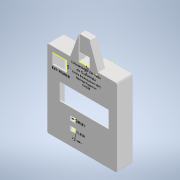
# Autodesk Inventor part: Cubierta SUperior
Saved by Autodesk Inventor 2021 (Build 250183000, 183)
## iProperties
Created: 2021-08-03
Part Number: Cubierta SUperior
Material: Generic
Document SubType Name: Modeling
Designer: Admin
Density: 1 g/cm^3
Appearance: Default
Author: Admin
Autodesk Inventor part; units mm, degrees
(part 1 of 3)
ref_plane "YZ Plane" through (0, 0, 0) normal (1, 0, 0) x (0, 1, 0)
ref_plane "XZ Plane" through (0, 0, 0) normal (0, 1, 0) x (-1, 0, 0)
ref_plane "XY Plane" through (0, 0, 0) normal (0, 0, 1) x (1, 0, 0)
sketch "Sketch1" plane through (0, 0, 0) normal (0, 0, 1) x (1, 0, 0)
  line L0 (-67.4504, -0.753) -> (-67.4504, -101.753) construction
  line L1 (24.2036, -1.253) -> (24.2036, -101.253) construction
  line L2 (24.2036, -101.253) -> (-64.9504, -101.253) construction
  line L3 (-64.9504, -101.253) -> (-64.9504, -1.253) construction
  line L4 (-64.9504, -1.253) -> (24.2036, -1.253) construction
  arc A0 (-65.4504, 1.247) -> (-67.4504, -0.753) centre (-65.4504, -0.753) ccw projected
  line L5 (-67.4504, -0.753) -> (-67.4504, -101.753) projected
  arc A1 (-67.4504, -101.753) -> (-65.4504, -103.753) centre (-65.4504, -101.753) ccw projected
  line L6 (-65.4504, -103.753) -> (26.7036, -103.753) projected
  line L7 (26.7036, -103.753) -> (26.7036, -0.753) projected
  arc A2 (26.7036, -0.753) -> (24.7036, 1.247) centre (24.7036, -0.753) ccw projected
  line L8 (24.7036, 1.247) -> (-65.4504, 1.247) projected
  line L9 (-52.1604, -58.503) -> (17.2396, -58.503) projected
  line L10 (17.2396, -58.503) -> (17.2396, -34.603) projected
  line L11 (17.2396, -34.603) -> (-52.1604, -34.603) projected
  line L12 (-52.1604, -34.603) -> (-52.1604, -58.503) projected
  line L13 (13.9003, -56.603) -> (-48.821, -56.603) projected
  arc A3 (14.3003, -57.003) -> (13.9003, -56.603) centre (13.9003, -57.003) ccw projected
  line L14 (14.3003, -57.203) -> (14.3003, -57.003) projected
  arc A4 (13.9003, -57.603) -> (14.3003, -57.203) centre (13.9003, -57.203) ccw projected
  line L15 (-48.821, -57.603) -> (13.9003, -57.603) projected
  arc A5 (-49.221, -57.203) -> (-48.821, -57.603) centre (-48.821, -57.203) ccw projected
  line L16 (-49.221, -57.003) -> (-49.221, -57.203) projected
  arc A6 (-48.821, -56.603) -> (-49.221, -57.003) centre (-48.821, -57.003) ccw projected
  line L17 (-49.221, -35.903) -> (-49.221, -36.103) projected
  arc A7 (-48.821, -35.503) -> (-49.221, -35.903) centre (-48.821, -35.903) ccw projected
  line L18 (13.9003, -35.503) -> (-48.821, -35.503) projected
  arc A8 (14.3003, -35.903) -> (13.9003, -35.503) centre (13.9003, -35.903) ccw projected
  line L19 (14.3003, -36.103) -> (14.3003, -35.903) projected
  arc A9 (13.9003, -36.503) -> (14.3003, -36.103) centre (13.9003, -36.103) ccw projected
  line L20 (-48.821, -36.503) -> (13.9003, -36.503) projected
  arc A10 (-49.221, -36.103) -> (-48.821, -36.503) centre (-48.821, -36.103) ccw projected
  line L21 (13.2396, -39.653) -> (-48.1604, -39.653) projected
  arc A11 (14.7396, -41.153) -> (13.2396, -39.653) centre (13.2396, -41.153) ccw projected
  line L22 (14.7396, -51.953) -> (14.7396, -41.153) projected
  arc A12 (13.2396, -53.453) -> (14.7396, -51.953) centre (13.2396, -51.953) ccw projected
  line L23 (-48.1604, -53.453) -> (13.2396, -53.453) projected
  arc A13 (-49.6604, -51.953) -> (-48.1604, -53.453) centre (-48.1604, -51.953) ccw projected
  line L24 (-49.6604, -41.153) -> (-49.6604, -51.953) projected
  arc A14 (-48.1604, -39.653) -> (-49.6604, -41.153) centre (-48.1604, -41.153) ccw projected
  arc A15 (-67.9504, 3.747) -> (-69.9504, 1.747) centre (-67.9504, 1.747) ccw projected
  line L25 (-67.9504, 3.747) -> (27.2036, 3.747) projected
  arc A16 (29.2036, 1.747) -> (27.2036, 3.747) centre (27.2036, 1.747) ccw projected
  line L26 (29.2036, 1.747) -> (29.2036, -104.253) projected
  arc A17 (27.2036, -106.253) -> (29.2036, -104.253) centre (27.2036, -104.253) ccw projected
  line L27 (27.2036, -106.253) -> (-67.9504, -106.253) projected
  arc A18 (-69.9504, -104.253) -> (-67.9504, -106.253) centre (-67.9504, -104.253) ccw projected
  line L28 (-69.9504, -104.253) -> (-69.9504, 1.747) projected
  circle A19 centre (-54.7104, -61.153) radius 1.7 construction
  circle A20 centre (-54.7104, -30.653) radius 1.7 construction
  circle A21 centre (19.7896, -61.153) radius 1.7 construction
  circle A22 centre (19.7896, -30.653) radius 1.7 construction
  line L29 (-64.9504, -101.253) -> (-64.9504, -1.253) projected
  line L30 (-64.9504, -1.253) -> (24.2036, -1.253) projected
  line L31 (24.2036, -1.253) -> (24.2036, -101.253) projected
  line L32 (24.2036, -101.253) -> (-64.9504, -101.253) projected
  line L33 (-74.9504, -109.253) -> (-74.9504, 6.747)
  arc A23 (-74.9504, -109.253) -> (-72.9504, -111.253) centre (-72.9504, -109.253) ccw
  line L34 (32.2036, -111.253) -> (-72.9504, -111.253)
  arc A24 (32.2036, -111.253) -> (34.2036, -109.253) centre (32.2036, -109.253) ccw
  line L35 (34.2036, 6.747) -> (34.2036, -109.253)
  arc A25 (34.2036, 6.747) -> (32.2036, 8.747) centre (32.2036, 6.747) ccw
  line L36 (-72.9504, 8.747) -> (32.2036, 8.747)
  arc A26 (-72.9504, 8.747) -> (-74.9504, 6.747) centre (-72.9504, 6.747) ccw
  point P0 (0, 0)
  constraints: 8 end point, 8 point on circle, 4 centre point, 2 horizontal, 2 vertical, 16 other
extrude "Extrusion1" add sketch "Sketch1" along normal blind 22.5 contours L25 A16 L26 A17 L27 A18 L28 A15
sketch "Sketch2" plane through (0, 0, 22.5) normal (0, 0, 1) x (1, 0, 0)
  line L0 (-52.1604, -58.503) -> (17.2396, -58.503) projected
  line L1 (17.2396, -58.503) -> (17.2396, -34.603) projected
  line L2 (17.2396, -34.603) -> (-52.1604, -34.603) projected
  line L3 (-52.1604, -34.603) -> (-52.1604, -58.503) projected
  line L4 (13.9003, -56.603) -> (-48.821, -56.603) projected
  arc A0 (14.3003, -57.003) -> (13.9003, -56.603) centre (13.9003, -57.003) ccw projected
  line L5 (14.3003, -57.203) -> (14.3003, -57.003) projected
  arc A1 (13.9003, -57.603) -> (14.3003, -57.203) centre (13.9003, -57.203) ccw projected
  line L6 (-48.821, -57.603) -> (13.9003, -57.603) projected
  arc A2 (-49.221, -57.203) -> (-48.821, -57.603) centre (-48.821, -57.203) ccw projected
  line L7 (-49.221, -57.003) -> (-49.221, -57.203) projected
  arc A3 (-48.821, -56.603) -> (-49.221, -57.003) centre (-48.821, -57.003) ccw projected
  line L8 (-49.221, -35.903) -> (-49.221, -36.103) projected
  arc A4 (-48.821, -35.503) -> (-49.221, -35.903) centre (-48.821, -35.903) ccw projected
  line L9 (13.9003, -35.503) -> (-48.821, -35.503) projected
  arc A5 (14.3003, -35.903) -> (13.9003, -35.503) centre (13.9003, -35.903) ccw projected
  line L10 (14.3003, -36.103) -> (14.3003, -35.903) projected
  arc A6 (13.9003, -36.503) -> (14.3003, -36.103) centre (13.9003, -36.103) ccw projected
  line L11 (-48.821, -36.503) -> (13.9003, -36.503) projected
  arc A7 (-49.221, -36.103) -> (-48.821, -36.503) centre (-48.821, -36.103) ccw projected
  line L12 (13.2396, -39.653) -> (-48.1604, -39.653) projected
  arc A8 (14.7396, -41.153) -> (13.2396, -39.653) centre (13.2396, -41.153) ccw projected
  line L13 (14.7396, -51.953) -> (14.7396, -41.153) projected
  arc A9 (13.2396, -53.453) -> (14.7396, -51.953) centre (13.2396, -51.953) ccw projected
  line L14 (-48.1604, -53.453) -> (13.2396, -53.453) projected
  arc A10 (-49.6604, -51.953) -> (-48.1604, -53.453) centre (-48.1604, -51.953) ccw projected
  line L15 (-49.6604, -41.153) -> (-49.6604, -51.953) projected
  arc A11 (-48.1604, -39.653) -> (-49.6604, -41.153) centre (-48.1604, -41.153) ccw projected
  line L16 (27.2036, 3.747) -> (-67.9504, 3.747) projected
  arc A12 (-67.9504, 3.747) -> (-69.9504, 1.747) centre (-67.9504, 1.747) ccw projected
  line L17 (-69.9504, 1.747) -> (-69.9504, -104.253) projected
  arc A13 (-69.9504, -104.253) -> (-67.9504, -106.253) centre (-67.9504, -104.253) ccw projected
  line L18 (-67.9504, -106.253) -> (27.2036, -106.253) projected
  arc A14 (27.2036, -106.253) -> (29.2036, -104.253) centre (27.2036, -104.253) ccw projected
  line L19 (29.2036, -104.253) -> (29.2036, 1.747) projected
  arc A15 (29.2036, 1.747) -> (27.2036, 3.747) centre (27.2036, 1.747) ccw projected
  line L20 (-35.8504, -70.273) -> (-35.8504, -73.173) construction
  line L21 (-35.8504, -73.173) -> (-31.8504, -73.173) construction
  line L22 (-31.8504, -73.173) -> (-31.8504, -70.273) construction
  line L23 (-31.8504, -70.273) -> (-35.8504, -70.273) construction
  circle A16 centre (-33.8504, -71.723) radius 0.875 construction
  line L24 (-31.8504, -85.773) -> (-31.8504, -82.873) construction
  line L25 (-31.8504, -82.873) -> (-35.8504, -82.873) construction
  line L26 (-35.8504, -82.873) -> (-35.8504, -85.773) construction
  line L27 (-35.8504, -85.773) -> (-31.8504, -85.773) construction
  circle A17 centre (-33.8504, -84.323) radius 0.875 construction
  line L28 (-37.3504, -68.773) -> (-37.3504, -74.673)
  line L29 (-37.3504, -74.673) -> (-30.3504, -74.673)
  line L30 (-30.3504, -74.673) -> (-30.3504, -68.773)
  line L31 (-30.3504, -68.773) -> (-37.3504, -68.773)
  line L32 (-37.3504, -81.373) -> (-30.3504, -81.373)
  line L33 (-30.3504, -81.373) -> (-30.3504, -87.273)
  line L34 (-30.3504, -87.273) -> (-37.3504, -87.273)
  line L35 (-37.3504, -87.273) -> (-37.3504, -81.373)
  point P0 (0, 0)
  dimension "d4" = 1.5
  dimension "d5" = 1.5
  constraints: 16 end point, 6 other
  measures "d4" distance between parallel lines of L31 L23
  measures "d5" distance between parallel lines of L32 L25
sketch "Sketch3" plane through (-67.9504, -106.253, 0) normal (0, -1, 0) x (1, 0, 0)
  line L0 (0, 0) -> (95.154, 0) construction
  line L1 (1.5, 20) -> (95.654, 20) construction
  line L2 (0, 22.5) -> (95.154, 22.5) construction
  line L3 (47.577, 22.5) -> (47.577, 0) construction
  line L4 (39.5436, 0) -> (55.4643, 0)
  line L5 (55.4643, 0) -> (55.4643, 6.6011)
  line L6 (55.4643, 6.6011) -> (39.5436, 6.6011)
  line L7 (39.5436, 6.6011) -> (39.5436, 0)
  line L8 (0, 0) -> (0, 22.5) projected
  point P0 (67.9504, 0)
  dimension "d6" = 39.5436
  dimension "d7" = 15.9207
  dimension "d8" = 13.3989
  constraints: 10 end point, 2 midpoint, 2 parallel, 1 horizontal, 1 perpendicular, 1 point on line
  measures "d6" distance between parallel lines of L8 L7
  measures "d7" distance of L5.end L6.end
  measures "d8" distance between parallel lines of L1 L6
extrude "Extrusion3" cut sketch "Sketch3" against normal blind 3
sketch "Sketch4" plane through (0, 0, 22.5) normal (0, 0, 1) x (1, 0, 0)
  line L0 (27.2036, 3.747) -> (-67.9504, 3.747) projected
  arc A0 (-67.9504, 3.747) -> (-69.9504, 1.747) centre (-67.9504, 1.747) ccw projected
  line L1 (-69.9504, 1.747) -> (-69.9504, -104.253) projected
  arc A1 (-69.9504, -104.253) -> (-67.9504, -106.253) centre (-67.9504, -104.253) ccw projected
  line L2 (-67.9504, -106.253) -> (27.2036, -106.253) projected
  arc A2 (27.2036, -106.253) -> (29.2036, -104.253) centre (27.2036, -104.253) ccw projected
  line L3 (29.2036, -104.253) -> (29.2036, 1.747) projected
  arc A3 (29.2036, 1.747) -> (27.2036, 3.747) centre (27.2036, 1.747) ccw projected
  line L4 (-65.4504, 1.247) -> (24.7036, 1.247) projected
  arc A4 (26.7036, -0.753) -> (24.7036, 1.247) centre (24.7036, -0.753) ccw projected
  line L5 (26.7036, -0.753) -> (26.7036, -103.753) projected
  line L6 (26.7036, -103.753) -> (-65.4504, -103.753) projected
  arc A5 (-67.4504, -101.753) -> (-65.4504, -103.753) centre (-65.4504, -101.753) ccw projected
  line L7 (-67.4504, -101.753) -> (-67.4504, -0.753) projected
  arc A6 (-65.4504, 1.247) -> (-67.4504, -0.753) centre (-65.4504, -0.753) ccw projected
  point P0 (0, 0)
extrude "Extrusion5" add sketch "Sketch4" against normal blind 2 contours L4 A4 L5 L6 A5 L7 A6
extrude "Extrusion4" cut sketch "Sketch2" against normal blind 12.25 contours L3 L2 L1 L0 | A0 L5 A1 L6 A2 L7 A3 L4 | A4 L9 A5 L10 A6 L11 A7 L8 | A8 L13 A9 L14 A10 L15 A11 L12 | L31 L30 L29 L28 | L32 L33 L34 L35
sketch "Sketch5" plane through (-67.9504, 3.747, 0) normal (0, 1, 0) x (1, 0, 0)
  point P0 (67.9504, 0)
sketch "Sketch6" plane through (-67.9504, 3.747, 0) normal (0, 1, 0) x (1, 0, 0)
  line L0 (58.24, -22.5) -> (42.74, -22.5)
  line L1 (42.74, -22.5) -> (42.74, -12.5)
  line L2 (42.74, -12.5) -> (58.24, -12.5)
  line L3 (58.24, -12.5) -> (58.24, -22.5)
  line L4 (15.79, -22.5) -> (85.19, -22.5) projected
  point P0 (67.9504, 0)
  point P1 (50.49, -22.5)
  point P2 (50.49, -22.5)
  dimension "d15" = 15.5
  dimension "d16" = 10
  constraints: 8 end point, 3 midpoint, 2 parallel, 1 coincident, 1 horizontal, 1 perpendicular
  measures "d15" distance of L1.end L2.end
  measures "d16" distance of L0.end L1.end
extrude "Extrusion6" add sketch "Sketch6" along normal blind 33
sketch "Sketch7" plane through (0, 0, 22.5) normal (0, 0, 1) x (1, 0, 0)
  line L0 (-25.2104, 36.747) -> (-9.7104, 36.747) projected
  line L1 (-9.7104, 36.747) -> (2.3007, 3.747)
  line L2 (27.2036, 3.747) -> (-67.9504, 3.747) projected
  line L3 (-25.2104, 3.747) -> (-25.2104, 36.747) projected
  line L4 (-25.2104, 36.747) -> (-37.2214, 3.747)
  line L5 (-25.2104, 3.747) -> (-67.9504, 3.747) projected
  line L6 (2.3007, 3.747) -> (-37.2214, 3.747)
  line L7 (-9.7104, 3.747) -> (-9.7104, 36.747) projected
  point P0 (0, 0)
  point P1 (-37.2214, 3.747)
  dimension "d19" = 20
  dimension "d20" = 20
  constraints: 6 end point, 2 point on line, 1 horizontal
  measures "d19" angle of L7 L1
  measures "d20" angle of L4 L3
extrude "Extrusion7" add sketch "Sketch7" against normal up to surface (10 mm away) contours L3 L2 L4 | L1 L2 L7
sketch "Sketch8" plane through (0, 0, 22.5) normal (0, 0, 1) x (1, 0, 0)
  line L0 (-25.2104, 36.747) -> (-9.7104, 36.747) projected
  line L1 (-9.7104, 36.747) -> (-9.7104, 3.747)
  line L2 (27.2036, 3.747) -> (-67.9504, 3.747) projected
  line L3 (-25.2002, 36.747) -> (-25.2002, 3.747)
  line L4 (-9.7104, 14.747) -> (-25.2002, 14.747)
  point P0 (0, 0)
  point P1 (-25.2002, 3.747)
  dimension "d23" = 15.4899
  dimension "d24" = 22
  constraints: 6 end point, 3 point on line, 2 vertical, 1 perpendicular
  measures "d23" distance between parallel lines of L3 L1
  measures "d24" distance between parallel lines of L0 L4
extrude "Extrusion8" cut sketch "Sketch8" against normal through all contours L4 L1 L2 L3
extrude "Extrusion9" cut sketch "Sketch8" against normal blind 1.5 contours L0 L1 L4 L3
sketch "Sketch9" plane through (-67.9504, 3.747, 0) normal (0, 1, 0) x (1, 0, 0)
  line L0 (57.577, -10) -> (37.577, -10)
  line L1 (37.577, -10) -> (37.577, 0)
  line L2 (37.577, 0) -> (57.577, 0)
  line L3 (57.577, 0) -> (57.577, -10)
  line L4 (95.154, 0) -> (0, 0) projected
  point P0 (67.9504, 0)
  point P1 (47.577, 0)
  point P2 (47.577, 0)
  dimension "d29" = 20
  dimension "d30" = 10
  constraints: 8 end point, 3 midpoint, 2 parallel, 1 coincident, 1 horizontal, 1 perpendicular
  measures "d29" distance of L0.start L0.end
  measures "d30" distance of L0.end L1.end
extrude "Extrusion10" cut sketch "Sketch9" against normal blind 71.25
sketch "Sketch10" plane through (0, 0, 22.5) normal (0, 0, 1) x (1, 0, 0)
  line L0 (-62.4504, -3.753) -> (-42.4504, -3.753)
  line L1 (-42.4504, -3.753) -> (-42.4504, -18.753)
  line L2 (-42.4504, -18.753) -> (-62.4504, -18.753)
  line L3 (-62.4504, -18.753) -> (-62.4504, -3.753)
  line L4 (-69.9504, 1.747) -> (-69.9504, -104.253) projected
  line L5 (-37.2214, 3.747) -> (-67.9504, 3.747) projected
  point P0 (0, 0)
  dimension "d33" = 20
  dimension "d34" = 15
  dimension "d35" = 7.5
  dimension "d36" = 7.5
  constraints: 8 end point, 2 parallel, 1 horizontal, 1 perpendicular
  measures "d33" distance of L1.end L2.end
  measures "d34" distance of L0.end L1.end
  measures "d35" distance between parallel lines of L4 L3
  measures "d36" distance between parallel lines of L5 L0
extrude "Extrusion11" cut sketch "Sketch10" against normal blind 10
sketch "Sketch11" plane through (0, 0, 22.5) normal (0, 0, 1) x (1, 0, 0)
  line L0 (-63.3072, -25.0311) -> (-40.5435, -25.0311) construction
  line L1 (-40.5435, -25.0311) -> (-40.5435, -19.9296) construction
  line L2 (-40.5435, -19.9296) -> (-63.3072, -19.9296) construction
  line L3 (-63.3072, -19.9296) -> (-63.3072, -25.0311) construction
  line L4 (-62.4504, -3.753) -> (-42.4504, -3.753) projected
  line L5 (-28.3504, -80.6683) -> (-5.5867, -80.6683) construction
  line L6 (-5.5867, -80.6683) -> (-5.5867, -62.7397) construction
  line L7 (-5.5867, -62.7397) -> (-28.3504, -62.7397) construction
  line L8 (-28.3504, -62.7397) -> (-28.3504, -80.6683) construction
  line L9 (-30.3504, -68.773) -> (-30.3504, -74.673) projected
  line L10 (-28.3504, -79.4502) -> (-28.3504, -97.3788) construction
  line L11 (-28.3504, -97.3788) -> (-5.2915, -97.3788) construction
  line L12 (-5.2915, -97.3788) -> (-5.2915, -79.4502) construction
  line L13 (-5.2915, -79.4502) -> (-28.3504, -79.4502) construction
  line L14 (-30.3504, -81.373) -> (-30.3504, -87.273) projected
  line L15 (-37.4504, -6.253) -> (8.5682, -6.253) construction
  line L16 (8.5682, -6.253) -> (8.5682, -17.71) construction
  line L17 (8.5682, -17.71) -> (-37.4504, -17.71) construction
  line L18 (-37.4504, -17.71) -> (-37.4504, -6.253) construction
  line L19 (-42.4504, -3.753) -> (-42.4504, -18.753) projected
  line L20 (-9.7104, 3.747) -> (-25.2002, 3.747) projected
  spline S0 degree 2 poles (-32.4935, -1.9798) (-32.4935, -3.2644) (-33.713, -3.2644) knots 0 0 0 1 1 1
  spline S1 degree 2 poles (-33.713, -3.2644) (-34.8786, -3.2644) (-34.8786, -2.0279) knots 0 0 0 1 1 1
  line L21 (-34.8786, -2.0279) -> (-34.8786, -0.1634)
  line L22 (-34.8786, -0.1634) -> (-34.3722, -0.1634)
  line L23 (-34.3722, -0.1634) -> (-34.3722, -1.9261)
  spline S2 degree 2 poles (-34.3722, -1.9261) (-34.3722, -2.823) (-33.6733, -2.823) knots 0 0 0 1 1 1
  spline S3 degree 2 poles (-33.6733, -2.823) (-33, -2.823) (-33, -1.9572) knots 0 0 0 1 1 1
  line L24 (-33, -1.9572) -> (-33, -0.1634)
  line L25 (-33, -0.1634) -> (-32.4935, -0.1634)
  line L26 (-32.4935, -0.1634) -> (-32.4935, -1.9798)
  line L27 (-29.8934, -3.2134) -> (-30.3857, -3.2134)
  line L28 (-30.3857, -3.2134) -> (-30.3857, -1.9855)
  spline S4 degree 2 poles (-30.3857, -1.9855) (-30.3857, -1.3744) (-30.8186, -1.3744) knots 0 0 0 1 1 1
  spline S5 degree 2 poles (-30.8186, -1.3744) (-31.0421, -1.3744) (-31.3363, -1.7139) (-31.3363, -1.9714) knots 0 0 0 1 2 2 2
  line L29 (-31.3363, -1.9714) -> (-31.3363, -3.2134)
  line L30 (-31.3363, -3.2134) -> (-31.8315, -3.2134)
  line L31 (-31.8315, -3.2134) -> (-31.8315, -1.0349)
  line L32 (-31.8315, -1.0349) -> (-31.3363, -1.0349)
  line L33 (-31.3363, -1.0349) -> (-31.3363, -1.397)
  line L34 (-31.3363, -1.397) -> (-31.3278, -1.397)
  spline S6 degree 2 poles (-31.3278, -1.397) (-31.0845, -0.9839) (-30.6233, -0.9839) knots 0 0 0 1 1 1
  spline S7 degree 2 poles (-30.6233, -0.9839) (-30.2668, -0.9839) (-29.8934, -1.4451) (-29.8934, -1.8808) knots 0 0 0 1 2 2 2
  line L35 (-29.8934, -1.8808) -> (-29.8934, -3.2134)
  line L36 (-28.7956, -3.2134) -> (-29.2879, -3.2134)
  line L37 (-29.2879, -3.2134) -> (-29.2879, -1.0349)
  line L38 (-29.2879, -1.0349) -> (-28.7956, -1.0349)
  line L39 (-28.7956, -1.0349) -> (-28.7956, -3.2134)
  spline S8 degree 2 poles (-29.0389, -0.5765) (-29.1606, -0.5765) (-29.3332, -0.4181) (-29.3332, -0.2964) knots 0 0 0 1 2 2 2
  spline S9 degree 2 poles (-29.3332, -0.2964) (-29.3332, -0.1747) (-29.1606, -0.0135) (-29.0389, -0.0135) knots 0 0 0 1 2 2 2
  spline S10 degree 2 poles (-29.0389, -0.0135) (-28.9144, -0.0135) (-28.739, -0.1747) (-28.739, -0.2964) knots 0 0 0 1 2 2 2
  spline S11 degree 2 poles (-28.739, -0.2964) (-28.739, -0.4124) (-28.9144, -0.5765) (-29.0389, -0.5765) knots 0 0 0 1 2 2 2
  line L40 (-26.2747, -1.0349) -> (-27.1178, -3.2134)
  line L41 (-27.1178, -3.2134) -> (-27.6526, -3.2134)
  line L42 (-27.6526, -3.2134) -> (-28.4533, -1.0349)
  line L43 (-28.4533, -1.0349) -> (-27.9185, -1.0349)
  line L44 (-27.9185, -1.0349) -> (-27.4347, -2.557)
  spline S12 degree 2 poles (-27.4347, -2.557) (-27.3781, -2.7268) (-27.3668, -2.8513) knots 0 0 0 1 1 1
  line L45 (-27.3668, -2.8513) -> (-27.3611, -2.8513)
  spline S13 degree 2 poles (-27.3611, -2.8513) (-27.3413, -2.6957) (-27.3017, -2.5655) knots 0 0 0 1 1 1
  line L46 (-27.3017, -2.5655) -> (-26.7953, -1.0349)
  line L47 (-26.7953, -1.0349) -> (-26.2747, -1.0349)
  line L48 (-24.0989, -2.2571) -> (-25.5815, -2.2571)
  spline S14 degree 2 poles (-25.5815, -2.2571) (-25.573, -2.5599) (-25.2194, -2.8881) (-24.9081, -2.8881) knots 0 0 0 1 2 2 2
  spline S15 degree 2 poles (-24.9081, -2.8881) (-24.5601, -2.8881) (-24.2687, -2.6787) knots 0 0 0 1 1 1
  line L49 (-24.2687, -2.6787) -> (-24.2687, -3.0776)
  spline S16 degree 2 poles (-24.2687, -3.0776) (-24.5658, -3.2644) (-25.0553, -3.2644) knots 0 0 0 1 1 1
  spline S17 degree 2 poles (-25.0553, -3.2644) (-25.5362, -3.2644) (-26.0823, -2.6702) (-26.0823, -2.1326) knots 0 0 0 1 2 2 2
  spline S18 degree 2 poles (-26.0823, -2.1326) (-26.0823, -1.6234) (-25.4797, -0.9839) (-25.0326, -0.9839) knots 0 0 0 1 2 2 2
  spline S19 degree 2 poles (-25.0326, -0.9839) (-24.5856, -0.9839) (-24.0989, -1.5583) (-24.0989, -2.0676) knots 0 0 0 1 2 2 2
  line L50 (-24.0989, -2.0676) -> (-24.0989, -2.2571)
  spline S20 degree 2 poles (-24.5743, -1.9091) (-24.5771, -1.6432) (-24.8233, -1.3489) (-25.0411, -1.3489) knots 0 0 0 1 2 2 2
  spline S21 degree 2 poles (-25.0411, -1.3489) (-25.2533, -1.3489) (-25.5476, -1.6573) (-25.5815, -1.9091) knots 0 0 0 1 2 2 2
  line L51 (-25.5815, -1.9091) -> (-24.5743, -1.9091)
  spline S22 degree 2 poles (-22.3646, -1.5045) (-22.4523, -1.4338) (-22.622, -1.4338) knots 0 0 0 1 1 1
  spline S23 degree 2 poles (-22.622, -1.4338) (-22.8399, -1.4338) (-23.1342, -1.8299) (-23.1342, -2.1694) knots 0 0 0 1 2 2 2
  line L52 (-23.1342, -2.1694) -> (-23.1342, -3.2134)
  line L53 (-23.1342, -3.2134) -> (-23.6265, -3.2134)
  line L54 (-23.6265, -3.2134) -> (-23.6265, -1.0349)
  line L55 (-23.6265, -1.0349) -> (-23.1342, -1.0349)
  line L56 (-23.1342, -1.0349) -> (-23.1342, -1.4819)
  line L57 (-23.1342, -1.4819) -> (-23.1257, -1.4819)
  spline S24 degree 2 poles (-23.1257, -1.4819) (-23.0521, -1.2527) (-22.7522, -0.9952) (-22.5683, -0.9952) knots 0 0 0 1 2 2 2
  spline S25 degree 2 poles (-22.5683, -0.9952) (-22.4353, -0.9952) (-22.3646, -1.0349) knots 0 0 0 1 1 1
  line L58 (-22.3646, -1.0349) -> (-22.3646, -1.5045)
  line L59 (-22.1524, -3.1455) -> (-22.1524, -2.69)
  spline S26 degree 2 poles (-22.1524, -2.69) (-21.8751, -2.8994) (-21.5412, -2.8994) knots 0 0 0 1 1 1
  spline S27 degree 2 poles (-21.5412, -2.8994) (-21.0942, -2.8994) (-21.0942, -2.6334) knots 0 0 0 1 1 1
  spline S28 degree 2 poles (-21.0942, -2.6334) (-21.0942, -2.5599) (-21.1706, -2.4552) (-21.3008, -2.376) (-21.4762, -2.3109) (-21.5865, -2.2713) knots 0 0 0 1 2 3 4 4 4
  spline S29 degree 2 poles (-21.5865, -2.2713) (-21.7195, -2.2175) (-21.9345, -2.0987) (-22.076, -1.9487) (-22.1495, -1.7563) (-22.1495, -1.629) knots 0 0 0 1 2 3 4 4 4
  spline S30 degree 2 poles (-22.1495, -1.629) (-22.1495, -1.4706) (-21.9996, -1.2301) (-21.7478, -1.066) (-21.4309, -0.9839) (-21.2611, -0.9839) knots 0 0 0 1 2 3 4 4 4
  spline S31 degree 2 poles (-21.2611, -0.9839) (-20.9584, -0.9839) (-20.7207, -1.0745) knots 0 0 0 1 1 1
  line L60 (-20.7207, -1.0745) -> (-20.7207, -1.5074)
  spline S32 degree 2 poles (-20.7207, -1.5074) (-20.9499, -1.3489) (-21.247, -1.3489) knots 0 0 0 1 1 1
  spline S33 degree 2 poles (-21.247, -1.3489) (-21.3404, -1.3489) (-21.4903, -1.3885) (-21.5978, -1.4564) (-21.6572, -1.5526) (-21.6572, -1.6092) knots 0 0 0 1 2 3 4 4 4
  spline S34 degree 2 poles (-21.6572, -1.6092) (-21.6572, -1.6799) (-21.5978, -1.7761) (-21.4818, -1.8525) (-21.3177, -1.9148) (-21.2102, -1.9487) knots 0 0 0 1 2 3 4 4 4
  spline S35 degree 2 poles (-21.2102, -1.9487) (-21.0716, -2.0081) (-20.8481, -2.127) (-20.6896, -2.2769) (-20.6047, -2.475) (-20.6047, -2.6108) knots 0 0 0 1 2 3 4 4 4
  spline S36 degree 2 poles (-20.6047, -2.6108) (-20.6047, -2.7777) (-20.7575, -3.0239) (-21.0122, -3.1851) (-21.346, -3.2644) (-21.5328, -3.2644) knots 0 0 0 1 2 3 4 4 4
  spline S37 degree 2 poles (-21.5328, -3.2644) (-21.8893, -3.2644) (-22.1524, -3.1455) knots 0 0 0 1 1 1
  line L61 (-19.6428, -3.2134) -> (-20.1351, -3.2134)
  line L62 (-20.1351, -3.2134) -> (-20.1351, -1.0349)
  line L63 (-20.1351, -1.0349) -> (-19.6428, -1.0349)
  line L64 (-19.6428, -1.0349) -> (-19.6428, -3.2134)
  spline S38 degree 2 poles (-19.8861, -0.5765) (-20.0078, -0.5765) (-20.1803, -0.4181) (-20.1803, -0.2964) knots 0 0 0 1 2 2 2
  spline S39 degree 2 poles (-20.1803, -0.2964) (-20.1803, -0.1747) (-20.0078, -0.0135) (-19.8861, -0.0135) knots 0 0 0 1 2 2 2
  spline S40 degree 2 poles (-19.8861, -0.0135) (-19.7616, -0.0135) (-19.5862, -0.1747) (-19.5862, -0.2964) knots 0 0 0 1 2 2 2
  spline S41 degree 2 poles (-19.5862, -0.2964) (-19.5862, -0.4124) (-19.7616, -0.5765) (-19.8861, -0.5765) knots 0 0 0 1 2 2 2
  line L65 (-17.0172, -3.2134) -> (-17.5123, -3.2134)
  line L66 (-17.5123, -3.2134) -> (-17.5123, -2.8428)
  line L67 (-17.5123, -2.8428) -> (-17.5208, -2.8428)
  spline S42 degree 2 poles (-17.5208, -2.8428) (-17.7585, -3.2644) (-18.2536, -3.2644) knots 0 0 0 1 1 1
  spline S43 degree 2 poles (-18.2536, -3.2644) (-18.6553, -3.2644) (-19.1392, -2.6787) (-19.1392, -2.1751) knots 0 0 0 1 2 2 2
  spline S44 degree 2 poles (-19.1392, -2.1751) (-19.1392, -1.6347) (-18.6044, -0.9839) (-18.1602, -0.9839) knots 0 0 0 1 2 2 2
  spline S45 degree 2 poles (-18.1602, -0.9839) (-17.7217, -0.9839) (-17.5208, -1.3376) knots 0 0 0 1 1 1
  line L68 (-17.5208, -1.3376) -> (-17.5123, -1.3376)
  line L69 (-17.5123, -1.3376) -> (-17.5123, 0.012)
  line L70 (-17.5123, 0.012) -> (-17.0172, 0.012)
  line L71 (-17.0172, 0.012) -> (-17.0172, -3.2134)
  line L72 (-17.5066, -2.2175) -> (-17.5066, -1.9317)
  spline S46 degree 2 poles (-17.5066, -1.9317) (-17.5066, -1.6997) (-17.8066, -1.3772) (-18.0414, -1.3772) knots 0 0 0 1 2 2 2
  spline S47 degree 2 poles (-18.0414, -1.3772) (-18.3187, -1.3772) (-18.6355, -1.7903) (-18.6355, -2.1553) knots 0 0 0 1 2 2 2
  spline S48 degree 2 poles (-18.6355, -2.1553) (-18.6355, -2.4891) (-18.33, -2.8739) (-18.0725, -2.8739) knots 0 0 0 1 2 2 2
  spline S49 degree 2 poles (-18.0725, -2.8739) (-17.8207, -2.8739) (-17.5066, -2.5004) (-17.5066, -2.2175) knots 0 0 0 1 2 2 2
  line L73 (-14.7, -3.2134) -> (-15.1809, -3.2134)
  line L74 (-15.1809, -3.2134) -> (-15.1809, -2.8739)
  line L75 (-15.1809, -2.8739) -> (-15.1894, -2.8739)
  spline S50 degree 2 poles (-15.1894, -2.8739) (-15.413, -3.2644) (-15.8487, -3.2644) knots 0 0 0 1 1 1
  spline S51 degree 2 poles (-15.8487, -3.2644) (-16.1712, -3.2644) (-16.5362, -2.9164) (-16.5362, -2.6278) knots 0 0 0 1 2 2 2
  spline S52 degree 2 poles (-16.5362, -2.6278) (-16.5362, -2.011) (-15.8232, -1.9091) knots 0 0 0 1 1 1
  line L76 (-15.8232, -1.9091) -> (-15.1781, -1.8186)
  spline S53 degree 2 poles (-15.1781, -1.8186) (-15.1781, -1.3517) (-15.6195, -1.3517) knots 0 0 0 1 1 1
  spline S54 degree 2 poles (-15.6195, -1.3517) (-16.0099, -1.3517) (-16.3212, -1.6205) knots 0 0 0 1 1 1
  line L77 (-16.3212, -1.6205) -> (-16.3212, -1.1876)
  spline S55 degree 2 poles (-16.3212, -1.1876) (-15.9788, -0.9839) (-15.5261, -0.9839) knots 0 0 0 1 1 1
  spline S56 degree 2 poles (-15.5261, -0.9839) (-14.7, -0.9839) (-14.7, -1.7959) knots 0 0 0 1 1 1
  line L78 (-14.7, -1.7959) -> (-14.7, -3.2134)
  line L79 (-15.1781, -2.1439) -> (-15.6365, -2.209)
  spline S57 degree 2 poles (-15.6365, -2.209) (-15.8487, -2.2345) (-16.0637, -2.3873) (-16.0637, -2.5768) knots 0 0 0 1 2 2 2
  spline S58 degree 2 poles (-16.0637, -2.5768) (-16.0637, -2.7155) (-15.8656, -2.8909) (-15.6987, -2.8909) knots 0 0 0 1 2 2 2
  spline S59 degree 2 poles (-15.6987, -2.8909) (-15.4724, -2.8909) (-15.1781, -2.574) (-15.1781, -2.3335) knots 0 0 0 1 2 2 2
  line L80 (-15.1781, -2.3335) -> (-15.1781, -2.1439)
  line L81 (-12.1168, -3.2134) -> (-12.6119, -3.2134)
  line L82 (-12.6119, -3.2134) -> (-12.6119, -2.8428)
  line L83 (-12.6119, -2.8428) -> (-12.6204, -2.8428)
  spline S60 degree 2 poles (-12.6204, -2.8428) (-12.8581, -3.2644) (-13.3532, -3.2644) knots 0 0 0 1 1 1
  spline S61 degree 2 poles (-13.3532, -3.2644) (-13.755, -3.2644) (-14.2388, -2.6787) (-14.2388, -2.1751) knots 0 0 0 1 2 2 2
  spline S62 degree 2 poles (-14.2388, -2.1751) (-14.2388, -1.6347) (-13.704, -0.9839) (-13.2598, -0.9839) knots 0 0 0 1 2 2 2
  spline S63 degree 2 poles (-13.2598, -0.9839) (-12.8213, -0.9839) (-12.6204, -1.3376) knots 0 0 0 1 1 1
  line L84 (-12.6204, -1.3376) -> (-12.6119, -1.3376)
  line L85 (-12.6119, -1.3376) -> (-12.6119, 0.012)
  line L86 (-12.6119, 0.012) -> (-12.1168, 0.012)
  line L87 (-12.1168, 0.012) -> (-12.1168, -3.2134)
  line L88 (-12.6063, -2.2175) -> (-12.6063, -1.9317)
  spline S64 degree 2 poles (-12.6063, -1.9317) (-12.6063, -1.6997) (-12.9062, -1.3772) (-13.141, -1.3772) knots 0 0 0 1 2 2 2
  spline S65 degree 2 poles (-13.141, -1.3772) (-13.4183, -1.3772) (-13.7352, -1.7903) (-13.7352, -2.1553) knots 0 0 0 1 2 2 2
  spline S66 degree 2 poles (-13.7352, -2.1553) (-13.7352, -2.4891) (-13.4296, -2.8739) (-13.1721, -2.8739) knots 0 0 0 1 2 2 2
  spline S67 degree 2 poles (-13.1721, -2.8739) (-12.9203, -2.8739) (-12.6063, -2.5004) (-12.6063, -2.2175) knots 0 0 0 1 2 2 2
  line L89 (-8.2944, -3.2134) -> (-8.7895, -3.2134)
  line L90 (-8.7895, -3.2134) -> (-8.7895, -2.8428)
  line L91 (-8.7895, -2.8428) -> (-8.798, -2.8428)
  spline S68 degree 2 poles (-8.798, -2.8428) (-9.0357, -3.2644) (-9.5308, -3.2644) knots 0 0 0 1 1 1
  spline S69 degree 2 poles (-9.5308, -3.2644) (-9.9326, -3.2644) (-10.4164, -2.6787) (-10.4164, -2.1751) knots 0 0 0 1 2 2 2
  spline S70 degree 2 poles (-10.4164, -2.1751) (-10.4164, -1.6347) (-9.8816, -0.9839) (-9.4374, -0.9839) knots 0 0 0 1 2 2 2
  spline S71 degree 2 poles (-9.4374, -0.9839) (-8.9989, -0.9839) (-8.798, -1.3376) knots 0 0 0 1 1 1
  line L92 (-8.798, -1.3376) -> (-8.7895, -1.3376)
  line L93 (-8.7895, -1.3376) -> (-8.7895, 0.012)
  line L94 (-8.7895, 0.012) -> (-8.2944, 0.012)
  line L95 (-8.2944, 0.012) -> (-8.2944, -3.2134)
  line L96 (-8.7839, -2.2175) -> (-8.7839, -1.9317)
  spline S72 degree 2 poles (-8.7839, -1.9317) (-8.7839, -1.6997) (-9.0838, -1.3772) (-9.3186, -1.3772) knots 0 0 0 1 2 2 2
  spline S73 degree 2 poles (-9.3186, -1.3772) (-9.5959, -1.3772) (-9.9128, -1.7903) (-9.9128, -2.1553) knots 0 0 0 1 2 2 2
  spline S74 degree 2 poles (-9.9128, -2.1553) (-9.9128, -2.4891) (-9.6072, -2.8739) (-9.3497, -2.8739) knots 0 0 0 1 2 2 2
  spline S75 degree 2 poles (-9.3497, -2.8739) (-9.0979, -2.8739) (-8.7839, -2.5004) (-8.7839, -2.2175) knots 0 0 0 1 2 2 2
  line L97 (-5.8074, -2.2571) -> (-7.29, -2.2571)
  spline S76 degree 2 poles (-7.29, -2.2571) (-7.2815, -2.5599) (-6.9278, -2.8881) (-6.6166, -2.8881) knots 0 0 0 1 2 2 2
  spline S77 degree 2 poles (-6.6166, -2.8881) (-6.2686, -2.8881) (-5.9772, -2.6787) knots 0 0 0 1 1 1
  line L98 (-5.9772, -2.6787) -> (-5.9772, -3.0776)
  spline S78 degree 2 poles (-5.9772, -3.0776) (-6.2743, -3.2644) (-6.7637, -3.2644) knots 0 0 0 1 1 1
  spline S79 degree 2 poles (-6.7637, -3.2644) (-7.2447, -3.2644) (-7.7908, -2.6702) (-7.7908, -2.1326) knots 0 0 0 1 2 2 2
  spline S80 degree 2 poles (-7.7908, -2.1326) (-7.7908, -1.6234) (-7.1881, -0.9839) (-6.7411, -0.9839) knots 0 0 0 1 2 2 2
  spline S81 degree 2 poles (-6.7411, -0.9839) (-6.2941, -0.9839) (-5.8074, -1.5583) (-5.8074, -2.0676) knots 0 0 0 1 2 2 2
  line L99 (-5.8074, -2.0676) -> (-5.8074, -2.2571)
  spline S82 degree 2 poles (-6.2828, -1.9091) (-6.2856, -1.6432) (-6.5317, -1.3489) (-6.7496, -1.3489) knots 0 0 0 1 2 2 2
  spline S83 degree 2 poles (-6.7496, -1.3489) (-6.9618, -1.3489) (-7.256, -1.6573) (-7.29, -1.9091) knots 0 0 0 1 2 2 2
  line L100 (-7.29, -1.9091) -> (-6.2828, -1.9091)
  line L101 (-4.8398, -3.2134) -> (-5.3349, -3.2134)
  line L102 (-5.3349, -3.2134) -> (-5.3349, 0.012)
  line L103 (-5.3349, 0.012) -> (-4.8398, 0.012)
  line L104 (-4.8398, 0.012) -> (-4.8398, -3.2134)
  line L105 (-0.5562, -0.1634) -> (-1.6512, -3.2134)
  line L106 (-1.6512, -3.2134) -> (-2.217, -3.2134)
  line L107 (-2.217, -3.2134) -> (-3.2922, -0.1634)
  line L108 (-3.2922, -0.1634) -> (-2.7405, -0.1634)
  line L109 (-2.7405, -0.1634) -> (-1.9879, -2.4778)
  spline S84 degree 2 poles (-1.9879, -2.4778) (-1.9511, -2.5881) (-1.9313, -2.7353) knots 0 0 0 1 1 1
  line L110 (-1.9313, -2.7353) -> (-1.9228, -2.7353)
  spline S85 degree 2 poles (-1.9228, -2.7353) (-1.9086, -2.6136) (-1.8605, -2.4721) knots 0 0 0 1 1 1
  line L111 (-1.8605, -2.4721) -> (-1.091, -0.1634)
  line L112 (-1.091, -0.1634) -> (-0.5562, -0.1634)
  line L113 (1.4667, -3.2134) -> (0.9857, -3.2134)
  line L114 (0.9857, -3.2134) -> (0.9857, -2.8739)
  line L115 (0.9857, -2.8739) -> (0.9773, -2.8739)
  spline S86 degree 2 poles (0.9773, -2.8739) (0.7537, -3.2644) (0.318, -3.2644) knots 0 0 0 1 1 1
  spline S87 degree 2 poles (0.318, -3.2644) (-0.0045, -3.2644) (-0.3695, -2.9164) (-0.3695, -2.6278) knots 0 0 0 1 2 2 2
  spline S88 degree 2 poles (-0.3695, -2.6278) (-0.3695, -2.011) (0.3435, -1.9091) knots 0 0 0 1 1 1
  line L116 (0.3435, -1.9091) -> (0.9886, -1.8186)
  spline S89 degree 2 poles (0.9886, -1.8186) (0.9886, -1.3517) (0.5472, -1.3517) knots 0 0 0 1 1 1
  spline S90 degree 2 poles (0.5472, -1.3517) (0.1568, -1.3517) (-0.1545, -1.6205) knots 0 0 0 1 1 1
  line L117 (-0.1545, -1.6205) -> (-0.1545, -1.1876)
  spline S91 degree 2 poles (-0.1545, -1.1876) (0.1879, -0.9839) (0.6406, -0.9839) knots 0 0 0 1 1 1
  spline S92 degree 2 poles (0.6406, -0.9839) (1.4667, -0.9839) (1.4667, -1.7959) knots 0 0 0 1 1 1
  line L118 (1.4667, -1.7959) -> (1.4667, -3.2134)
  line L119 (0.9886, -2.1439) -> (0.5302, -2.209)
  spline S93 degree 2 poles (0.5302, -2.209) (0.318, -2.2345) (0.103, -2.3873) (0.103, -2.5768) knots 0 0 0 1 2 2 2
  spline S94 degree 2 poles (0.103, -2.5768) (0.103, -2.7155) (0.3011, -2.8909) (0.468, -2.8909) knots 0 0 0 1 2 2 2
  spline S95 degree 2 poles (0.468, -2.8909) (0.6943, -2.8909) (0.9886, -2.574) (0.9886, -2.3335) knots 0 0 0 1 2 2 2
  line L120 (0.9886, -2.3335) -> (0.9886, -2.1439)
  line L121 (2.5645, -3.2134) -> (2.0694, -3.2134)
  line L122 (2.0694, -3.2134) -> (2.0694, 0.012)
  line L123 (2.0694, 0.012) -> (2.5645, 0.012)
  line L124 (2.5645, 0.012) -> (2.5645, -3.2134)
  line L125 (3.7019, -3.2134) -> (3.2068, -3.2134)
  line L126 (3.2068, -3.2134) -> (3.2068, 0.012)
  line L127 (3.2068, 0.012) -> (3.7019, 0.012)
  line L128 (3.7019, 0.012) -> (3.7019, -3.2134)
  line L129 (6.186, -2.2571) -> (4.7035, -2.2571)
  spline S96 degree 2 poles (4.7035, -2.2571) (4.712, -2.5599) (5.0656, -2.8881) (5.3768, -2.8881) knots 0 0 0 1 2 2 2
  spline S97 degree 2 poles (5.3768, -2.8881) (5.7248, -2.8881) (6.0163, -2.6787) knots 0 0 0 1 1 1
  line L130 (6.0163, -2.6787) -> (6.0163, -3.0776)
  spline S98 degree 2 poles (6.0163, -3.0776) (5.7192, -3.2644) (5.2297, -3.2644) knots 0 0 0 1 1 1
  spline S99 degree 2 poles (5.2297, -3.2644) (4.7487, -3.2644) (4.2027, -2.6702) (4.2027, -2.1326) knots 0 0 0 1 2 2 2
  spline S100 degree 2 poles (4.2027, -2.1326) (4.2027, -1.6234) (4.8053, -0.9839) (5.2524, -0.9839) knots 0 0 0 1 2 2 2
  spline S101 degree 2 poles (5.2524, -0.9839) (5.6994, -0.9839) (6.186, -1.5583) (6.186, -2.0676) knots 0 0 0 1 2 2 2
  line L131 (6.186, -2.0676) -> (6.186, -2.2571)
  spline S102 degree 2 poles (5.7107, -1.9091) (5.7079, -1.6432) (5.4617, -1.3489) (5.2439, -1.3489) knots 0 0 0 1 2 2 2
  spline S103 degree 2 poles (5.2439, -1.3489) (5.0317, -1.3489) (4.7374, -1.6573) (4.7035, -1.9091) knots 0 0 0 1 2 2 2
  line L132 (4.7035, -1.9091) -> (5.7107, -1.9091)
  line L133 (-25.8517, -9.0655) -> (-26.3468, -9.0655)
  line L134 (-26.3468, -9.0655) -> (-26.3468, -8.6949)
  line L135 (-26.3468, -8.6949) -> (-26.3553, -8.6949)
  spline S104 degree 2 poles (-26.3553, -8.6949) (-26.593, -9.1164) (-27.0881, -9.1164) knots 0 0 0 1 1 1
  spline S105 degree 2 poles (-27.0881, -9.1164) (-27.4899, -9.1164) (-27.9737, -8.5308) (-27.9737, -8.0272) knots 0 0 0 1 2 2 2
  spline S106 degree 2 poles (-27.9737, -8.0272) (-27.9737, -7.4868) (-27.439, -6.836) (-26.9947, -6.836) knots 0 0 0 1 2 2 2
  spline S107 degree 2 poles (-26.9947, -6.836) (-26.5562, -6.836) (-26.3553, -7.1897) knots 0 0 0 1 1 1
  line L136 (-26.3553, -7.1897) -> (-26.3468, -7.1897)
  line L137 (-26.3468, -7.1897) -> (-26.3468, -5.8401)
  line L138 (-26.3468, -5.8401) -> (-25.8517, -5.8401)
  line L139 (-25.8517, -5.8401) -> (-25.8517, -9.0655)
  line L140 (-26.3412, -8.0696) -> (-26.3412, -7.7838)
  spline S108 degree 2 poles (-26.3412, -7.7838) (-26.3412, -7.5518) (-26.6411, -7.2293) (-26.8759, -7.2293) knots 0 0 0 1 2 2 2
  spline S109 degree 2 poles (-26.8759, -7.2293) (-27.1532, -7.2293) (-27.4701, -7.6424) (-27.4701, -8.0074) knots 0 0 0 1 2 2 2
  spline S110 degree 2 poles (-27.4701, -8.0074) (-27.4701, -8.3412) (-27.1645, -8.726) (-26.907, -8.726) knots 0 0 0 1 2 2 2
  spline S111 degree 2 poles (-26.907, -8.726) (-26.6552, -8.726) (-26.3412, -8.3525) (-26.3412, -8.0696) knots 0 0 0 1 2 2 2
  line L141 (-23.3647, -8.1092) -> (-24.8473, -8.1092)
  spline S112 degree 2 poles (-24.8473, -8.1092) (-24.8388, -8.4119) (-24.4851, -8.7401) (-24.1739, -8.7401) knots 0 0 0 1 2 2 2
  spline S113 degree 2 poles (-24.1739, -8.7401) (-23.8259, -8.7401) (-23.5345, -8.5308) knots 0 0 0 1 1 1
  line L142 (-23.5345, -8.5308) -> (-23.5345, -8.9297)
  spline S114 degree 2 poles (-23.5345, -8.9297) (-23.8316, -9.1164) (-24.321, -9.1164) knots 0 0 0 1 1 1
  spline S115 degree 2 poles (-24.321, -9.1164) (-24.802, -9.1164) (-25.3481, -8.5223) (-25.3481, -7.9847) knots 0 0 0 1 2 2 2
  spline S116 degree 2 poles (-25.3481, -7.9847) (-25.3481, -7.4754) (-24.7454, -6.836) (-24.2984, -6.836) knots 0 0 0 1 2 2 2
  spline S117 degree 2 poles (-24.2984, -6.836) (-23.8514, -6.836) (-23.3647, -7.4104) (-23.3647, -7.9196) knots 0 0 0 1 2 2 2
  line L143 (-23.3647, -7.9196) -> (-23.3647, -8.1092)
  spline S118 degree 2 poles (-23.8401, -7.7612) (-23.8429, -7.4952) (-24.089, -7.201) (-24.3069, -7.201) knots 0 0 0 1 2 2 2
  spline S119 degree 2 poles (-24.3069, -7.201) (-24.5191, -7.201) (-24.8133, -7.5094) (-24.8473, -7.7612) knots 0 0 0 1 2 2 2
  line L144 (-24.8473, -7.7612) -> (-23.8401, -7.7612)
  spline S120 degree 2 poles (-19.2594, -8.8561) (-19.7376, -9.1164) (-20.3232, -9.1164) knots 0 0 0 1 1 1
  spline S121 degree 2 poles (-20.3232, -9.1164) (-20.9994, -9.1164) (-21.8369, -8.2733) (-21.8369, -7.5801) knots 0 0 0 1 2 2 2
  spline S122 degree 2 poles (-21.8369, -7.5801) (-21.8369, -6.8728) (-20.9202, -5.9646) (-20.2129, -5.9646) knots 0 0 0 1 2 2 2
  spline S123 degree 2 poles (-20.2129, -5.9646) (-19.7064, -5.9646) (-19.3584, -6.1145) knots 0 0 0 1 1 1
  line L145 (-19.3584, -6.1145) -> (-19.3584, -6.6351)
  spline S124 degree 2 poles (-19.3584, -6.6351) (-19.7093, -6.4003) (-20.1959, -6.4003) knots 0 0 0 1 1 1
  spline S125 degree 2 poles (-20.1959, -6.4003) (-20.6825, -6.4003) (-21.305, -7.0426) (-21.305, -7.5547) knots 0 0 0 1 2 2 2
  spline S126 degree 2 poles (-21.305, -7.5547) (-21.305, -8.0781) (-20.7703, -8.6807) (-20.3091, -8.6807) knots 0 0 0 1 2 2 2
  spline S127 degree 2 poles (-20.3091, -8.6807) (-19.995, -8.6807) (-19.7659, -8.5591) knots 0 0 0 1 1 1
  line L146 (-19.7659, -8.5591) -> (-19.7659, -7.8319)
  line L147 (-19.7659, -7.8319) -> (-20.4081, -7.8319)
  line L148 (-20.4081, -7.8319) -> (-20.4081, -7.4075)
  line L149 (-20.4081, -7.4075) -> (-19.2594, -7.4075)
  line L150 (-19.2594, -7.4075) -> (-19.2594, -8.8561)
  line L151 (-16.7583, -9.0655) -> (-17.2506, -9.0655)
  line L152 (-17.2506, -9.0655) -> (-17.2506, -8.7203)
  line L153 (-17.2506, -8.7203) -> (-17.2591, -8.7203)
  spline S128 degree 2 poles (-17.2591, -8.7203) (-17.4741, -9.1164) (-17.9296, -9.1164) knots 0 0 0 1 1 1
  spline S129 degree 2 poles (-17.9296, -9.1164) (-18.6992, -9.1164) (-18.6992, -8.1884) knots 0 0 0 1 1 1
  line L154 (-18.6992, -8.1884) -> (-18.6992, -6.8869)
  line L155 (-18.6992, -6.8869) -> (-18.2069, -6.8869)
  line L156 (-18.2069, -6.8869) -> (-18.2069, -8.1375)
  spline S130 degree 2 poles (-18.2069, -8.1375) (-18.2069, -8.726) (-17.7542, -8.726) knots 0 0 0 1 1 1
  spline S131 degree 2 poles (-17.7542, -8.726) (-17.5335, -8.726) (-17.2506, -8.4035) (-17.2506, -8.1403) knots 0 0 0 1 2 2 2
  line L157 (-17.2506, -8.1403) -> (-17.2506, -6.8869)
  line L158 (-17.2506, -6.8869) -> (-16.7583, -6.8869)
  line L159 (-16.7583, -6.8869) -> (-16.7583, -9.0655)
  line L160 (-14.4411, -9.0655) -> (-14.9221, -9.0655)
  line L161 (-14.9221, -9.0655) -> (-14.9221, -8.726)
  line L162 (-14.9221, -8.726) -> (-14.9306, -8.726)
  spline S132 degree 2 poles (-14.9306, -8.726) (-15.1541, -9.1164) (-15.5898, -9.1164) knots 0 0 0 1 1 1
  spline S133 degree 2 poles (-15.5898, -9.1164) (-15.9123, -9.1164) (-16.2773, -8.7684) (-16.2773, -8.4798) knots 0 0 0 1 2 2 2
  spline S134 degree 2 poles (-16.2773, -8.4798) (-16.2773, -7.8631) (-15.5643, -7.7612) knots 0 0 0 1 1 1
  line L163 (-15.5643, -7.7612) -> (-14.9192, -7.6707)
  spline S135 degree 2 poles (-14.9192, -7.6707) (-14.9192, -7.2038) (-15.3606, -7.2038) knots 0 0 0 1 1 1
  spline S136 degree 2 poles (-15.3606, -7.2038) (-15.7511, -7.2038) (-16.0623, -7.4726) knots 0 0 0 1 1 1
  line L164 (-16.0623, -7.4726) -> (-16.0623, -7.0397)
  spline S137 degree 2 poles (-16.0623, -7.0397) (-15.7199, -6.836) (-15.2672, -6.836) knots 0 0 0 1 1 1
  spline S138 degree 2 poles (-15.2672, -6.836) (-14.4411, -6.836) (-14.4411, -7.648) knots 0 0 0 1 1 1
  line L165 (-14.4411, -7.648) -> (-14.4411, -9.0655)
  line L166 (-14.9192, -7.996) -> (-15.3776, -8.0611)
  spline S139 degree 2 poles (-15.3776, -8.0611) (-15.5898, -8.0866) (-15.8048, -8.2394) (-15.8048, -8.4289) knots 0 0 0 1 2 2 2
  spline S140 degree 2 poles (-15.8048, -8.4289) (-15.8048, -8.5676) (-15.6068, -8.743) (-15.4398, -8.743) knots 0 0 0 1 2 2 2
  spline S141 degree 2 poles (-15.4398, -8.743) (-15.2135, -8.743) (-14.9192, -8.4261) (-14.9192, -8.1856) knots 0 0 0 1 2 2 2
  line L167 (-14.9192, -8.1856) -> (-14.9192, -7.996)
  spline S142 degree 2 poles (-12.6897, -9.0401) (-12.8369, -9.1136) (-13.0717, -9.1136) knots 0 0 0 1 1 1
  spline S143 degree 2 poles (-13.0717, -9.1136) (-13.7055, -9.1136) (-13.7055, -8.5053) knots 0 0 0 1 1 1
  line L168 (-13.7055, -8.5053) -> (-13.7055, -7.2746)
  line L169 (-13.7055, -7.2746) -> (-14.0704, -7.2746)
  line L170 (-14.0704, -7.2746) -> (-14.0704, -6.8869)
  line L171 (-14.0704, -6.8869) -> (-13.7055, -6.8869)
  line L172 (-13.7055, -6.8869) -> (-13.7055, -6.3833)
  line L173 (-13.7055, -6.3833) -> (-13.2132, -6.2419)
  line L174 (-13.2132, -6.2419) -> (-13.2132, -6.8869)
  line L175 (-13.2132, -6.8869) -> (-12.6897, -6.8869)
  line L176 (-12.6897, -6.8869) -> (-12.6897, -7.2746)
  line L177 (-12.6897, -7.2746) -> (-13.2132, -7.2746)
  line L178 (-13.2132, -7.2746) -> (-13.2132, -8.3638)
  spline S144 degree 2 poles (-13.2132, -8.3638) (-13.2132, -8.5562) (-13.0717, -8.7232) (-12.9076, -8.7232) knots 0 0 0 1 2 2 2
  spline S145 degree 2 poles (-12.9076, -8.7232) (-12.7831, -8.7232) (-12.6897, -8.6496) knots 0 0 0 1 1 1
  line L179 (-12.6897, -8.6496) -> (-12.6897, -9.0401)
  line L180 (-10.4235, -8.1092) -> (-11.906, -8.1092)
  spline S146 degree 2 poles (-11.906, -8.1092) (-11.8975, -8.4119) (-11.5439, -8.7401) (-11.2326, -8.7401) knots 0 0 0 1 2 2 2
  spline S147 degree 2 poles (-11.2326, -8.7401) (-10.8846, -8.7401) (-10.5932, -8.5308) knots 0 0 0 1 1 1
  line L181 (-10.5932, -8.5308) -> (-10.5932, -8.9297)
  spline S148 degree 2 poles (-10.5932, -8.9297) (-10.8903, -9.1164) (-11.3798, -9.1164) knots 0 0 0 1 1 1
  spline S149 degree 2 poles (-11.3798, -9.1164) (-11.8607, -9.1164) (-12.4068, -8.5223) (-12.4068, -7.9847) knots 0 0 0 1 2 2 2
  spline S150 degree 2 poles (-12.4068, -7.9847) (-12.4068, -7.4754) (-11.8042, -6.836) (-11.3571, -6.836) knots 0 0 0 1 2 2 2
  spline S151 degree 2 poles (-11.3571, -6.836) (-10.9101, -6.836) (-10.4235, -7.4104) (-10.4235, -7.9196) knots 0 0 0 1 2 2 2
  line L182 (-10.4235, -7.9196) -> (-10.4235, -8.1092)
  spline S152 degree 2 poles (-10.8988, -7.7612) (-10.9016, -7.4952) (-11.1478, -7.201) (-11.3656, -7.201) knots 0 0 0 1 2 2 2
  spline S153 degree 2 poles (-11.3656, -7.201) (-11.5778, -7.201) (-11.8721, -7.5094) (-11.906, -7.7612) knots 0 0 0 1 2 2 2
  line L183 (-11.906, -7.7612) -> (-10.8988, -7.7612)
  line L184 (-6.6944, -9.0655) -> (-7.1867, -9.0655)
  line L185 (-7.1867, -9.0655) -> (-7.1867, -7.8772)
  spline S154 degree 2 poles (-7.1867, -7.8772) (-7.1867, -7.5349) (-7.3819, -7.2293) (-7.6111, -7.2293) knots 0 0 0 1 2 2 2
  spline S155 degree 2 poles (-7.6111, -7.2293) (-7.8035, -7.2293) (-8.0751, -7.6169) (-8.0751, -7.8857) knots 0 0 0 1 2 2 2
  line L186 (-8.0751, -7.8857) -> (-8.0751, -9.0655)
  line L187 (-8.0751, -9.0655) -> (-8.5703, -9.0655)
  line L188 (-8.5703, -9.0655) -> (-8.5703, -7.8376)
  spline S156 degree 2 poles (-8.5703, -7.8376) (-8.5703, -7.2293) (-9.0003, -7.2293) knots 0 0 0 1 1 1
  spline S157 degree 2 poles (-9.0003, -7.2293) (-9.2012, -7.2293) (-9.4587, -7.5943) (-9.4587, -7.8857) knots 0 0 0 1 2 2 2
  line L189 (-9.4587, -7.8857) -> (-9.4587, -9.0655)
  line L190 (-9.4587, -9.0655) -> (-9.951, -9.0655)
  line L191 (-9.951, -9.0655) -> (-9.951, -6.8869)
  line L192 (-9.951, -6.8869) -> (-9.4587, -6.8869)
  line L193 (-9.4587, -6.8869) -> (-9.4587, -7.2321)
  line L194 (-9.4587, -7.2321) -> (-9.4502, -7.2321)
  spline S158 degree 2 poles (-9.4502, -7.2321) (-9.2125, -6.836) (-8.7627, -6.836) knots 0 0 0 1 1 1
  spline S159 degree 2 poles (-8.7627, -6.836) (-8.5363, -6.836) (-8.1996, -7.085) (-8.1374, -7.2859) knots 0 0 0 1 2 2 2
  spline S160 degree 2 poles (-8.1374, -7.2859) (-7.8941, -6.836) (-7.4131, -6.836) knots 0 0 0 1 1 1
  spline S161 degree 2 poles (-7.4131, -6.836) (-6.6944, -6.836) (-6.6944, -7.7244) knots 0 0 0 1 1 1
  line L195 (-6.6944, -7.7244) -> (-6.6944, -9.0655)
  line L196 (-4.4197, -9.0655) -> (-4.9006, -9.0655)
  line L197 (-4.9006, -9.0655) -> (-4.9006, -8.726)
  line L198 (-4.9006, -8.726) -> (-4.9091, -8.726)
  spline S162 degree 2 poles (-4.9091, -8.726) (-5.1326, -9.1164) (-5.5684, -9.1164) knots 0 0 0 1 1 1
  spline S163 degree 2 poles (-5.5684, -9.1164) (-5.8909, -9.1164) (-6.2559, -8.7684) (-6.2559, -8.4798) knots 0 0 0 1 2 2 2
  spline S164 degree 2 poles (-6.2559, -8.4798) (-6.2559, -7.8631) (-5.5429, -7.7612) knots 0 0 0 1 1 1
  line L199 (-5.5429, -7.7612) -> (-4.8978, -7.6707)
  spline S165 degree 2 poles (-4.8978, -7.6707) (-4.8978, -7.2038) (-5.3392, -7.2038) knots 0 0 0 1 1 1
  spline S166 degree 2 poles (-5.3392, -7.2038) (-5.7296, -7.2038) (-6.0409, -7.4726) knots 0 0 0 1 1 1
  line L200 (-6.0409, -7.4726) -> (-6.0409, -7.0397)
  spline S167 degree 2 poles (-6.0409, -7.0397) (-5.6985, -6.836) (-5.2458, -6.836) knots 0 0 0 1 1 1
  spline S168 degree 2 poles (-5.2458, -6.836) (-4.4197, -6.836) (-4.4197, -7.648) knots 0 0 0 1 1 1
  line L201 (-4.4197, -7.648) -> (-4.4197, -9.0655)
  line L202 (-4.8978, -7.996) -> (-5.3562, -8.0611)
  spline S169 degree 2 poles (-5.3562, -8.0611) (-5.5684, -8.0866) (-5.7834, -8.2394) (-5.7834, -8.4289) knots 0 0 0 1 2 2 2
  spline S170 degree 2 poles (-5.7834, -8.4289) (-5.7834, -8.5676) (-5.5853, -8.743) (-5.4184, -8.743) knots 0 0 0 1 2 2 2
  spline S171 degree 2 poles (-5.4184, -8.743) (-5.1921, -8.743) (-4.8978, -8.4261) (-4.8978, -8.1856) knots 0 0 0 1 2 2 2
  line L203 (-4.8978, -8.1856) -> (-4.8978, -7.996)
  line L204 (-3.3219, -9.0655) -> (-3.817, -9.0655)
  line L205 (-3.817, -9.0655) -> (-3.817, -5.8401)
  line L206 (-3.817, -5.8401) -> (-3.3219, -5.8401)
  line L207 (-3.3219, -5.8401) -> (-3.3219, -9.0655)
  line L208 (-1.0075, -9.0655) -> (-1.4885, -9.0655)
  line L209 (-1.4885, -9.0655) -> (-1.4885, -8.726)
  line L210 (-1.4885, -8.726) -> (-1.497, -8.726)
  spline S172 degree 2 poles (-1.497, -8.726) (-1.7205, -9.1164) (-2.1562, -9.1164) knots 0 0 0 1 1 1
  spline S173 degree 2 poles (-2.1562, -9.1164) (-2.4787, -9.1164) (-2.8437, -8.7684) (-2.8437, -8.4798) knots 0 0 0 1 2 2 2
  spline S174 degree 2 poles (-2.8437, -8.4798) (-2.8437, -7.8631) (-2.1307, -7.7612) knots 0 0 0 1 1 1
  line L211 (-2.1307, -7.7612) -> (-1.4857, -7.6707)
  spline S175 degree 2 poles (-1.4857, -7.6707) (-1.4857, -7.2038) (-1.927, -7.2038) knots 0 0 0 1 1 1
  spline S176 degree 2 poles (-1.927, -7.2038) (-2.3175, -7.2038) (-2.6287, -7.4726) knots 0 0 0 1 1 1
  line L212 (-2.6287, -7.4726) -> (-2.6287, -7.0397)
  spline S177 degree 2 poles (-2.6287, -7.0397) (-2.2864, -6.836) (-1.8337, -6.836) knots 0 0 0 1 1 1
  spline S178 degree 2 poles (-1.8337, -6.836) (-1.0075, -6.836) (-1.0075, -7.648) knots 0 0 0 1 1 1
  line L213 (-1.0075, -7.648) -> (-1.0075, -9.0655)
  line L214 (-1.4857, -7.996) -> (-1.944, -8.0611)
  spline S179 degree 2 poles (-1.944, -8.0611) (-2.1562, -8.0866) (-2.3712, -8.2394) (-2.3712, -8.4289) knots 0 0 0 1 2 2 2
  spline S180 degree 2 poles (-2.3712, -8.4289) (-2.3712, -8.5676) (-2.1732, -8.743) (-2.0063, -8.743) knots 0 0 0 1 2 2 2
  spline S181 degree 2 poles (-2.0063, -8.743) (-1.7799, -8.743) (-1.4857, -8.4261) (-1.4857, -8.1856) knots 0 0 0 1 2 2 2
  line L215 (-1.4857, -8.1856) -> (-1.4857, -7.996)
  line L216 (-32.5592, -11.6431) -> (-33.4711, -14.1831)
  line L217 (-33.4711, -14.1831) -> (-33.9423, -14.1831)
  line L218 (-33.9423, -14.1831) -> (-34.8377, -11.6431)
  line L219 (-34.8377, -11.6431) -> (-34.3782, -11.6431)
  line L220 (-34.3782, -11.6431) -> (-33.7514, -13.5705)
  spline S182 degree 2 poles (-33.7514, -13.5705) (-33.7208, -13.6624) (-33.7043, -13.7849) knots 0 0 0 1 1 1
  line L221 (-33.7043, -13.7849) -> (-33.6973, -13.7849)
  spline S183 degree 2 poles (-33.6973, -13.7849) (-33.6855, -13.6836) (-33.6454, -13.5658) knots 0 0 0 1 1 1
  line L222 (-33.6454, -13.5658) -> (-33.0045, -11.6431)
  line L223 (-33.0045, -11.6431) -> (-32.5592, -11.6431)
  line L224 (-30.8745, -14.1831) -> (-31.2751, -14.1831)
  line L225 (-31.2751, -14.1831) -> (-31.2751, -13.9004)
  line L226 (-31.2751, -13.9004) -> (-31.2821, -13.9004)
  spline S184 degree 2 poles (-31.2821, -13.9004) (-31.4683, -14.2255) (-31.8311, -14.2255) knots 0 0 0 1 1 1
  spline S185 degree 2 poles (-31.8311, -14.2255) (-32.0997, -14.2255) (-32.4037, -13.9357) (-32.4037, -13.6954) knots 0 0 0 1 2 2 2
  spline S186 degree 2 poles (-32.4037, -13.6954) (-32.4037, -13.1817) (-31.8099, -13.0969) knots 0 0 0 1 1 1
  line L227 (-31.8099, -13.0969) -> (-31.2727, -13.0215)
  spline S187 degree 2 poles (-31.2727, -13.0215) (-31.2727, -12.6327) (-31.6403, -12.6327) knots 0 0 0 1 1 1
  spline S188 degree 2 poles (-31.6403, -12.6327) (-31.9654, -12.6327) (-32.2246, -12.8566) knots 0 0 0 1 1 1
  line L228 (-32.2246, -12.8566) -> (-32.2246, -12.496)
  spline S189 degree 2 poles (-32.2246, -12.496) (-31.9395, -12.3264) (-31.5625, -12.3264) knots 0 0 0 1 1 1
  spline S190 degree 2 poles (-31.5625, -12.3264) (-30.8745, -12.3264) (-30.8745, -13.0026) knots 0 0 0 1 1 1
  line L229 (-30.8745, -13.0026) -> (-30.8745, -14.1831)
  line L230 (-31.2727, -13.2925) -> (-31.6544, -13.3466)